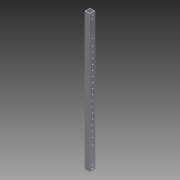
# Autodesk Inventor part: Chassis V1.500 Part2
Saved by Autodesk Inventor 2013 (Build 170138000, 138)
## iProperties
Created: 2013-01-05
Part Number: Chassis V1.500 Part2
Material: Aluminum 6061
Document SubType Name: Modeling
Designer: Moses
Density: 2.71 g/cm^3
Mass: 493.363 g
Surface Area: 1178.78 cm^2
Volume: 182.053 cm^3
Author: Moses
Autodesk Inventor part; units mm, degrees
ref_plane "YZ Plane" through (0, 0, 0) normal (1, 0, 0) x (0, 1, 0)
ref_plane "XZ Plane" through (0, 0, 0) normal (0, 1, 0) x (-1, 0, 0)
ref_plane "XY Plane" through (0, 0, 0) normal (0, 0, 1) x (1, 0, 0)
sketch "Sketch1" plane through (0, 0, 0) normal (0, 1, 0) x (-1, 0, 0)
  line L0 (0, 25.4) -> (25.4, 25.4)
  line L1 (25.4, 25.4) -> (25.4, 0)
  line L2 (25.4, 0) -> (0, 0)
  line L3 (0, 0) -> (0, 25.4)
  line L4 (22.225, 22.225) -> (3.175, 22.225)
  line L5 (3.175, 22.225) -> (3.175, 3.175)
  line L6 (3.175, 3.175) -> (22.225, 3.175)
  line L7 (22.225, 3.175) -> (22.225, 22.225)
  dimension "d0" = 25.4
  dimension "d1" = 25.4
  dimension "d2" = 3.175
  constraints: 16 end point, 4 parallel, 2 perpendicular, 1 coincident, 1 horizontal, 3 other
  measures "d0" distance of L1.end L2.end
  measures "d1" distance of L0.end L1.end
  measures "d2" distance between parallel lines of L0 L4
extrude "Extrusion1" add sketch "Sketch1" along normal blind 660.4
sketch "Sketch2" plane through (-25.4, 0, 25.4) normal (0, 0, 1) x (1, 0, 0)
  line L0 (25.4, 0) -> (0, 0) projected
  line L1 (0, 660.4) -> (25.4, 660.4) projected
  line L2 (12.7, 660.4) -> (12.7, 0) construction
  circle A0 centre (12.7, 50.8) radius 2.8575
  circle A1 centre (12.7, 88.0533) radius 2.8575
  circle A2 centre (12.7, 125.3067) radius 2.8575
  circle A3 centre (12.7, 162.56) radius 2.8575
  circle A4 centre (12.7, 199.8133) radius 2.8575
  circle A5 centre (12.7, 237.0667) radius 2.8575
  circle A6 centre (12.7, 274.32) radius 2.8575
  circle A7 centre (12.7, 311.5733) radius 2.8575
  circle A8 centre (12.7, 348.8267) radius 2.8575
  circle A9 centre (12.7, 386.08) radius 2.8575
  circle A10 centre (12.7, 423.3333) radius 2.8575
  circle A11 centre (12.7, 460.5867) radius 2.8575
  circle A12 centre (12.7, 497.84) radius 2.8575
  circle A13 centre (12.7, 535.0933) radius 2.8575
  circle A14 centre (12.7, 572.3467) radius 2.8575
  circle A15 centre (12.7, 609.6) radius 2.8575
  dimension "d5" = 5.715
  dimension "d6" = 50.8
  dimension "d7" = 660.4
  dimension "d10" = 37.2533
  constraints: 16 centre point, 2 end point, 2 midpoint, 1 point on line, 1 vertical, 30 other
  measures "d5" diameter of A0
  measures "d6" distance from line of L0 A0.centre
  measures "d7" distance of L0.end L1.start
  measures "d10" distance of A0.centre A1.centre
extrude "Extrusion2" [suppressed]
sketch "Sketch3" plane through (-25.4, 0, 0) normal (-1, 0, 0) x (0, 0, 1)
  line L0 (25.4, 0) -> (0, 0) projected
  line L1 (0, 660.4) -> (25.4, 660.4) projected
  line L2 (12.7, 660.4) -> (12.7, 0) construction
  circle A0 centre (12.7, 552.45) radius 3.302
  circle A1 centre (12.7, 107.95) radius 3.302
  circle A2 centre (12.7, 650.875) radius 3.302 projected
  circle A3 centre (12.7, 635) radius 3.302 projected
  circle A4 centre (12.7, 25.4) radius 3.302 projected
  circle A5 centre (12.7, 9.525) radius 3.302 projected
  circle A6 centre (12.7, 520.7) radius 3.302
  circle A7 centre (12.7, 495.3) radius 3.302
  circle A8 centre (12.7, 469.9) radius 3.302
  circle A9 centre (12.7, 444.5) radius 3.302
  circle A10 centre (12.7, 419.1) radius 3.302
  circle A11 centre (12.7, 393.7) radius 3.302
  circle A12 centre (12.7, 368.3) radius 3.302
  circle A13 centre (12.7, 342.9) radius 3.302
  circle A14 centre (12.7, 317.5) radius 3.302
  circle A15 centre (12.7, 292.1) radius 3.302
  circle A16 centre (12.7, 266.7) radius 3.302
  circle A17 centre (12.7, 241.3) radius 3.302
  circle A18 centre (12.7, 215.9) radius 3.302
  circle A19 centre (12.7, 190.5) radius 3.302
  circle A20 centre (12.7, 165.1) radius 3.302
  circle A21 centre (12.7, 139.7) radius 3.302
  dimension "d27" = 6.604
  dimension "d28" = 6.604
  dimension "d29" = 107.95
  dimension "d30" = 107.95
  dimension "d31" = 444.5
  dimension "d32" = 31.75
  dimension "d33" = 6.604
  dimension "d36" = 25.4
  constraints: 18 centre point, 3 point on line, 2 end point, 2 midpoint, 1 vertical, 30 other
  measures "d27" diameter of A1
  measures "d28" diameter of A0
  measures "d29" distance from line of L1 A0.centre
  measures "d30" distance from line of L0 A1.centre
  measures "d31" distance of A1.centre A0.centre
  measures "d32" distance of A6.centre A0.centre
  measures "d33" diameter of A6
  measures "d36" distance of A6.centre A7.centre
extrude "Extrusion3" cut sketch "Sketch3" against normal blind 25.4
equation "\"d27\" = d28"
equation "\"d30\" = d29"
equation "\"d33\" = d28"
body "Solid1"
